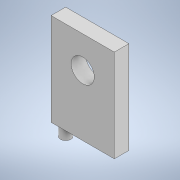
# Autodesk Inventor part: Spring connection
Saved by Autodesk Inventor 2021 (Build 250183000, 183)
## iProperties
Created: 2020-10-21
Part Number: Spring connection
Material: Generic
Document SubType Name: Modeling
Designer: nabee
Density: 1 g/cm^3
Appearance: Default
Author: nabee
Autodesk Inventor part; units mm, degrees
ref_plane "YZ Plane" through (0, 0, 0) normal (1, 0, 0) x (0, 1, 0)
ref_plane "XZ Plane" through (0, 0, 0) normal (0, 1, 0) x (-1, 0, 0)
ref_plane "XY Plane" through (0, 0, 0) normal (0, 0, 1) x (1, 0, 0)
sketch "Sketch9" plane through (0, 0, 0) normal (0, 0, 1) x (1, 0, 0)
  line L0 (0, 0) -> (130, 0)
  line L1 (130, 0) -> (130, 130)
  line L2 (130, 130) -> (0, 130)
  line L3 (0, 130) -> (0, 0)
  dimension "d32" = 130
  dimension "d33" = 130
  constraints: 8 end point, 2 parallel, 1 horizontal, 1 perpendicular
  measures "d32" distance of L0.start L0.end
  measures "d33" distance of L2.end L0.start
extrude "Extrusion9" add sketch "Sketch9" along normal blind 30
sketch "Sketch10" plane through (0, 0, 30) normal (0, 0, 1) x (1, 0, 0)
  line L0 (0, 130) -> (0, 0) projected
  line L1 (130, 0) -> (130, 130) projected
  line L2 (0, 130) -> (130, 0) construction
  circle A0 centre (65, 65) radius 23.8125
  dimension "d36" = 47.625
  constraints: 2 end point, 1 centre point, 1 midpoint
  measures "d36" diameter of A0
extrude "Extrusion10" cut sketch "Sketch10" against normal blind 40
sketch "Sketch11" plane through (0, 0, 0) normal (-1, 0, 0) x (0, 0, 1)
  point P0 (0, 0)
sketch "Sketch12" plane through (0, 0, 0) normal (0, -1, 0) x (1, 0, 0)
  line L0 (130, 0) -> (130, 30) projected
  line L1 (0, 0) -> (130, 0)
  line L2 (130, 0) -> (130, 30)
  line L3 (130, 30) -> (0, 30)
  line L4 (0, 30) -> (0, 0)
  constraints: 8 end point, 2 parallel, 1 horizontal, 1 perpendicular
extrude "Extrusion11" add sketch "Sketch12" along normal blind 40
sketch "Sketch13" plane through (0, -40, 0) normal (0, -1, 0) x (1, 0, 0)
  line L0 (130, 30) -> (0, 30) projected
  line L1 (0, 0) -> (130, 0)
  line L2 (130, 0) -> (130, 30)
  line L3 (130, 30) -> (0, 30)
  line L4 (0, 30) -> (0, 0)
  point P0 (0, 30)
  constraints: 8 end point, 2 parallel, 1 horizontal, 1 perpendicular
extrude "Extrusion12" cut sketch "Sketch13" against normal blind 20
sketch "Sketch15" plane through (0, -20, 0) normal (0, -1, 0) x (1, 0, 0)
  line L0 (130, 30) -> (0, 30) projected
  line L1 (130, 30) -> (0, 30)
  line L2 (0, 30) -> (0, 0)
  line L3 (0, 0) -> (130, 0)
  line L4 (130, 0) -> (130, 30)
  point P0 (0, 30)
  constraints: 8 end point, 2 parallel, 1 horizontal, 1 perpendicular
extrude "Extrusion14" add sketch "Sketch15" along normal blind 40
sketch "Sketch16" plane through (0, -60, 0) normal (0, -1, 0) x (1, 0, 0)
  line L0 (130, 30) -> (0, 30) projected
  line L1 (130, 30) -> (0, 30)
  line L2 (0, 30) -> (0, 0)
  line L3 (0, 0) -> (130, 0)
  line L4 (130, 0) -> (130, 30)
  constraints: 8 end point, 2 parallel, 1 horizontal, 1 perpendicular
extrude "Extrusion15" cut sketch "Sketch16" against normal blind 15
sketch "Sketch17" plane through (0, -45, 0) normal (0, -1, 0) x (1, 0, 0)
  line L0 (130, 30) -> (0, 30) projected
  line L1 (130, 30) -> (0, 30)
  line L2 (0, 30) -> (0, 0)
  line L3 (0, 0) -> (130, 0)
  line L4 (130, 0) -> (130, 30)
  constraints: 8 end point, 2 parallel, 1 horizontal, 1 perpendicular
extrude "Extrusion16" cut sketch "Sketch17" against normal blind 10
sketch "Sketch19" plane through (0, -35, 0) normal (0, -1, 0) x (1, 0, 0)
  circle A0 centre (25, 15) radius 10.682
  line L0 (0, 30) -> (130, 30) projected
  line L1 (0, 0) -> (0, 30) projected
  dimension "d64" = 21.364
  dimension "d65" = 15
  dimension "d66" = 25
  constraints: 1 centre point
  measures "d64" diameter of A0
  measures "d65" distance from line of L0 A0.centre
  measures "d66" distance from line of L1 A0.centre
extrude "Extrusion18" add sketch "Sketch19" along normal blind 15
sketch "Sketch20" plane through (0, -35, 0) normal (0, -1, 0) x (1, 0, 0)
  line L0 (0, 0) -> (0, 30) projected
  line L1 (0, 30) -> (130, 30) projected
  line L2 (0, 0) -> (130, 0)
  line L3 (130, 0) -> (130, 30)
  line L4 (130, 30) -> (0, 30)
  line L5 (0, 30) -> (0, 0)
  constraints: 8 end point, 2 parallel, 1 horizontal, 1 perpendicular
extrude "Extrusion19" add sketch "Sketch20" along normal blind 25
sketch "Sketch21" plane through (0, -60, 0) normal (0, -1, 0) x (1, 0, 0)
  circle A0 centre (15, 15) radius 10.682
  line L0 (130, 30) -> (0, 30) projected
  line L1 (0, 30) -> (0, 0) projected
  dimension "d71" = 21.364
  dimension "d72" = 15
  dimension "d73" = 15
  constraints: 1 centre point
  measures "d71" diameter of A0
  measures "d72" distance from line of L0 A0.centre
  measures "d73" distance from line of L1 A0.centre
extrude "Extrusion20" add sketch "Sketch21" along normal blind 25
body "Solid2"
